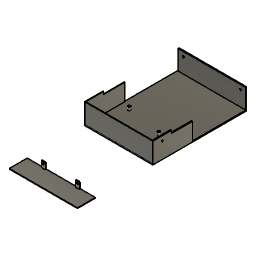
BakjeCNCPCBShizzle v1 (Autodesk Fusion 360 design; units mm, degrees)
Autodesk Fusion 360 part; units mm, degrees
sketch "Sketch1" plane through (0, 0, 0) normal (0, 0, 1) x (1, 0, 0)
  line L0 (0, 142.5) -> (129, 142.5)
  line L1 (129, 142.5) -> (129, 217.5)
  line L2 (129, 217.5) -> (0, 217.5)
  line L3 (0, 217.5) -> (0, 142.5)
  line L4 (0, 0) -> (1, 0)
  line L5 (1, 217.5) -> (0, 217.5)
  line L6 (129, 217.5) -> (0, 217.5)
  line L7 (0, 217.5) -> (0, 320)
  line L8 (0, 320) -> (129, 320)
  line L9 (129, 320) -> (129, 217.5)
  line L10 (0, 217.5) -> (1, 217.5)
  line L11 (1, 217.5) -> (1, 142.5)
  line L12 (1, 142.5) -> (0, 142.5)
  line L13 (0, 142.5) -> (0, 217.5)
  line L14 (129, 142.5) -> (127, 142.5)
  line L15 (127, 142.5) -> (127, 217.5)
  line L16 (127, 217.5) -> (129, 217.5)
  line L17 (129, 217.5) -> (129, 142.5)
  line L18 (0, 320) -> (129, 320)
  line L19 (129, 320) -> (129, 318)
  line L20 (129, 318) -> (0, 318)
  line L21 (0, 318) -> (0, 320)
  line L22 (1, 142.5) -> (127, 142.5)
  line L23 (127, 142.5) -> (127, 143.5)
  line L24 (127, 143.5) -> (1, 143.5)
  line L25 (1, 143.5) -> (1, 142.5)
  line L26 (0, 320) -> (1, 320)
  line L27 (1, 320) -> (1, 283)
  line L28 (1, 283) -> (0, 283)
  line L29 (0, 283) -> (0, 320)
  line L30 (0, 217.5) -> (0, 177.5)
  line L31 (0, 177.5) -> (1, 177.5)
  line L32 (1, 177.5) -> (129, 177.5)
  dimension "d2" = 142.5
  dimension "d3" = 129
  dimension "d4" = 75
  dimension "d5" = 1
  dimension "d6" = 129
  dimension "d7" = 102.5
  dimension "d8" = 1
  dimension "d9" = 2
  dimension "d10" = 2
  dimension "d11" = 1
  dimension "d12" = 1
  dimension "d29" = 40
  constraint horizontal L0
  constraint vertical L1
  constraint horizontal L2
  constraint vertical L3
  constraint horizontal L4
  constraint horizontal L5
  constraint coincident L2 L5.start
  constraint coincident L4.start origin
  constraint horizontal L6
  constraint vertical L7
  constraint horizontal L8
  constraint vertical L9
  constraint horizontal L10
  constraint vertical L11
  constraint horizontal L12
  constraint vertical L13
  constraint horizontal L14
  constraint vertical L15
  constraint horizontal L16
  constraint vertical L17
  constraint coincident L6 L15.end
  constraint horizontal L18
  constraint vertical L19
  constraint horizontal L20
  constraint vertical L21
  constraint coincident L9 L19.end
  constraint horizontal L22
  constraint vertical L23
  constraint horizontal L24
  constraint vertical L25
  constraint horizontal L26
  constraint vertical L27
  constraint horizontal L28
  constraint vertical L29
  constraint coincident L3 L30.end
  constraint coincident L11 L31.end
  constraint perpendicular L11 L31
  constraint coincident L17 L32.end
  constraint perpendicular L17 L32
  measures "d2" distance of L4.start L0.start
  measures "d3" distance of L0.start L0.end
  measures "d4" distance of L0.start L2.end
  measures "d5" distance of L4.start L4.end
  measures "d6" distance of L1.end L2.end
  measures "d7" distance of L1.end L8.end
  measures "d8" distance of L2.end L5.start
  measures "d9" distance of L0.end L14.end
  measures "d10" distance of L7.end L20.end
  measures "d11" distance of L11.end L24.end
  measures "d12" distance of L7.end L26.end
  measures "d29" distance of L2.end L30.end
extrude "Extrude1" add sketch "Sketch1" along normal blind 39 contours L0 L3 L11 L12 L13 L25 L31 | L0 L11 L15 L22 L23 L24 L25 | L0 L1 L14 L15 L17 L23 L32 | L8 L9 L18 L19 L20 L27 makes body 1 at (43.6667, 320, 13) makes body 2 at (43, 142.5, 26)
extrude "Extrude2" add sketch "Sketch1" along normal blind 2 contours L11 L15 L24 L32 | L2 L5 L6 L7 L9 L10 L16 L20 L27 L28 | L2 L6 L11 L15 L32 | L7 L20 L27 L28 L29 bodies 1 2
sketch "Sketch2" plane through (0, 318, 0) normal (0, -1, 0) x (1, 0, 0)
  line L0 (1, 2) -> (129, 2)
  line L1 (129, 2) -> (129, 39)
  line L2 (129, 39) -> (1, 39)
  line L3 (1, 39) -> (1, 2)
  line L4 (1, 39) -> (129, 39)
  line L5 (1, 39) -> (11, 39)
  line L6 (11, 39) -> (11, 30.25)
  circle A0 centre (11, 30.25) radius 1.75
  line L7 (129, 39) -> (119, 39)
  line L8 (119, 39) -> (119, 30.25)
  circle A1 centre (119, 30.25) radius 1.75
  dimension "d17" = 10
  dimension "d18" = 8.75
  dimension "d19" = 3.5
  dimension "d20" = 10
  dimension "d21" = 8.75
  dimension "d22" = 3.5
  constraint coincident L2.end L3.start
  constraint coincident L1.end L2.start
  constraint perpendicular L3 L5
  constraint perpendicular L5 L6
  constraint coincident L6.end A0.centre
  constraint perpendicular L1 L7
  constraint perpendicular L7 L8
  constraint coincident L8.end A1.centre
  measures "d17" distance of L2.end L5.end
  measures "d18" distance of L5.end L6.end
  measures "d19" diameter of A0
  measures "d20" distance of L1.end L7.end
  measures "d21" distance of L7.end L8.end
  measures "d22" diameter of A1
extrude "Extrude3" cut sketch "Sketch2" against normal blind 90 contours A0 | A1 bodies 1
sketch "Sketch3" plane through (127, 0, 0) normal (-1, 0, 0) x (0, -1, 0)
  line L0 (-177.5, 2) -> (-143.5, 2)
  line L1 (-143.5, 2) -> (-143.5, 39)
  line L2 (-143.5, 39) -> (-177.5, 39)
  line L3 (-177.5, 39) -> (-143.5, 39)
  line L4 (-160.5, 39) -> (-160.5, 30.25)
  circle A0 centre (-160.5, 30.25) radius 1.75
  line L5 (-177.5, 39) -> (-177.5, 2)
  dimension "d25" = 8.75
  dimension "d26" = 3.5
  constraint coincident L2.end L3.start
  constraint coincident L1.end L2.start
  constraint midpoint L3 L4.start
  constraint perpendicular L3 L4
  constraint coincident L4.end A0.centre
  measures "d25" distance of L4.start L4.end
  measures "d26" diameter of A0
extrude "Extrude4" cut sketch "Sketch3" against normal blind 43 contours A0 bodies 1
sketch "Sketch4" plane through (0, 0, 2) normal (0, 0, 1) x (-1, 0, 0)
  line L0 (-129, -318) -> (-1, -318)
  line L1 (-1, -318) -> (0, -318)
  line L2 (0, -318) -> (0, -217.5)
  line L3 (-129, -217.5) -> (-129, -318)
  line L4 (0, -217.5) -> (-1, -217.5)
  line L5 (-127, -217.5) -> (-129, -217.5)
  line L6 (-1, -217.5) -> (-1, -177.5)
  line L7 (-1, -177.5) -> (-1, -143.5)
  line L8 (-1, -143.5) -> (-127, -143.5)
  line L9 (-127, -143.5) -> (-127, -177.5)
  line L10 (-127, -177.5) -> (-127, -217.5)
extrude "Extrude5" add sketch "Sketch1" along normal blind 34 contours L2 L3 L5 L6 L10 L11 L13 L30 L31 | L1 L2 L6 L15 L16 L17 L32 bodies 1
sketch "Sketch5" plane through (0, 0, 0) normal (0, 0, 1) x (1, 0, 0)
  line L0 (0, 0) -> (129, 0)
  line L1 (129, 0) -> (129, 34)
  line L2 (129, 34) -> (0, 34)
  line L3 (0, 34) -> (0, 0)
  line L4 (0, 34) -> (129, 34)
  line L5 (64.5, 34) -> (0, 34)
  line L6 (64.5, 34) -> (129, 34)
  line L7 (32.25, 34) -> (32.25, 33)
  line L8 (96.75, 34) -> (96.75, 33)
  line L9 (36, 34) -> (28.5, 34)
  line L10 (28.5, 34) -> (28.5, 32)
  line L11 (28.5, 32) -> (36, 32)
  line L12 (36, 32) -> (36, 34)
  line L13 (36, 34) -> (28.5, 32) construction
  line L14 (28.5, 34) -> (36, 32) construction
  line L15 (100.5, 32) -> (93, 32)
  line L16 (93, 32) -> (93, 34)
  line L17 (93, 34) -> (100.5, 34)
  line L18 (100.5, 34) -> (100.5, 32)
  line L19 (100.5, 32) -> (93, 34) construction
  line L20 (93, 32) -> (100.5, 34) construction
  point P0 (32.25, 33)
  point P1 (96.75, 33)
  dimension "d32" = 129
  dimension "d33" = 34
  dimension "d34" = 1
  dimension "d35" = 1
  dimension "d36" = 7.5
  dimension "d37" = 2
  dimension "d38" = 7.5
  dimension "d39" = 2
  constraint horizontal L0
  constraint vertical L1
  constraint horizontal L2
  constraint vertical L3
  constraint coincident L0.start L3.end
  constraint midpoint L2 L5.start
  constraint midpoint L5 L7.start
  constraint perpendicular L4 L7
  constraint midpoint L6 L8.start
  constraint vertical L8
  constraint horizontal L9
  constraint perpendicular L9 L10
  constraint parallel L9 L11
  constraint parallel L10 L12
  constraint coincident L13 P0
  constraint coincident L14 P0
  constraint coincident P0 L7.end
  constraint horizontal L15
  constraint perpendicular L15 L16
  constraint parallel L15 L17
  constraint parallel L16 L18
  constraint coincident L19 P1
  constraint coincident L20 P1
  constraint coincident P1 L8.end
  measures "d32" distance of L0.start L0.end
  measures "d33" distance of L0.start L2.end
  measures "d34" distance of L7.start P0
  measures "d35" distance of L8.start P1
  measures "d36" distance of L10.end L11.end
  measures "d37" distance of L9.end L10.end
  measures "d38" distance of L16.end L17.end
  measures "d39" distance of L15.end L16.end
extrude "Extrude6" add sketch "Sketch5" along normal blind 1 separate body contours L0 L1 L2 L3 L4 L5 L6 L10 L11 L12 L15 L16 L18 makes body 3
extrude "Extrude7" add sketch "Sketch5" along normal blind 12.25 contours L2 L4 L5 L9 L10 L11 L12 | L2 L4 L6 L15 L16 L17 L18 bodies 3
sketch "Sketch6" plane through (0, 32, 0) normal (0, -1, 0) x (1, 0, 0)
  line L0 (28.5, 1) -> (36, 1)
  line L1 (36, 1) -> (36, 12.25)
  line L2 (36, 12.25) -> (28.5, 12.25)
  line L3 (28.5, 12.25) -> (28.5, 1)
  line L4 (32.25, 1) -> (32.25, 8.75)
  circle A0 centre (32.25, 8.75) radius 1.75
  dimension "d44" = 7.75
  dimension "d45" = 3.5
  constraint midpoint L0 L4.start
  constraint perpendicular L0 L4
  constraint coincident L4.end A0.centre
  measures "d44" distance of L4.start L4.end
  measures "d45" diameter of A0
sketch "Sketch7" plane through (0, 32, 0) normal (0, -1, 0) x (1, 0, 0)
  line L0 (93, 1) -> (100.5, 1)
  line L1 (100.5, 1) -> (100.5, 12.25)
  line L2 (100.5, 12.25) -> (93, 12.25)
  line L3 (93, 12.25) -> (93, 1)
  line L4 (96.75, 1) -> (96.75, 8.75)
  circle A0 centre (96.75, 8.75) radius 1.75
  dimension "d46" = 7.75
  dimension "d47" = 3.5
  constraint midpoint L0 L4.start
  constraint perpendicular L0 L4
  constraint coincident L4.end A0.centre
  measures "d46" distance of L4.start L4.end
  measures "d47" diameter of A0
extrude "Extrude8" cut sketch "Sketch6" sketch "Sketch7" against normal blind 15 contours A0 of sketch 2 contours A0 bodies 3
sketch "Sketch8" plane through (0, 0, 2) normal (0, 0, 1) x (-1, 0, 0)
  line L0 (-127, -217.5) -> (-129, -217.5)
  line L1 (-129, -217.5) -> (-129, -318)
  line L2 (-129, -318) -> (-1, -318)
  line L3 (-1, -318) -> (0, -318)
  line L4 (0, -318) -> (0, -217.5)
  line L5 (0, -217.5) -> (-1, -217.5)
  line L6 (-1, -217.5) -> (-1, -143.5)
  line L7 (-1, -143.5) -> (-127, -143.5)
  line L8 (-127, -143.5) -> (-127, -217.5)
  line L9 (-127, -217.5) -> (-1, -217.5)
  line L10 (-64, -217.5) -> (-64, -143.5)
  line L11 (-64, -217.5) -> (-127, -217.5)
  line L12 (-95.5, -217.5) -> (-95.5, -143.5)
  line L13 (-127, -217.5) -> (-95.5, -143.5)
  line L14 (-100.25, -159.5) -> (-122.25, -159.5)
  line L15 (-122.25, -159.5) -> (-122.25, -201.5)
  line L16 (-122.25, -201.5) -> (-100.25, -201.5)
  line L17 (-100.25, -201.5) -> (-100.25, -159.5)
  line L18 (-100.25, -159.5) -> (-122.25, -201.5) construction
  line L19 (-122.25, -159.5) -> (-100.25, -201.5) construction
  line L20 (-64, -143.5) -> (-95.5, -217.5)
  line L21 (-68.75, -201.5) -> (-90.75, -201.5)
  line L22 (-90.75, -201.5) -> (-90.75, -159.5)
  line L23 (-90.75, -159.5) -> (-68.75, -159.5)
  line L24 (-68.75, -159.5) -> (-68.75, -201.5)
  line L25 (-68.75, -201.5) -> (-90.75, -159.5) construction
  line L26 (-90.75, -201.5) -> (-68.75, -159.5) construction
  line L27 (-100.25, -159.5) -> (-100.25, -166)
  line L28 (-100.25, -166) -> (-103.25, -166)
  circle A0 centre (-103.25, -166) radius 1.5
  line L29 (-122.25, -201.5) -> (-122.25, -195)
  line L30 (-122.25, -195) -> (-119.25, -195)
  circle A1 centre (-103.25, -166) radius 2.5
  circle A2 centre (-119.25, -195) radius 1.5
  circle A3 centre (-119.25, -195) radius 2.5
  line L31 (-68.75, -159.5) -> (-68.75, -166)
  line L32 (-68.75, -166) -> (-71.75, -166)
  circle A4 centre (-71.75, -166) radius 1.5
  circle A5 centre (-71.75, -166) radius 2.5
  line L33 (-90.75, -201.5) -> (-90.75, -195)
  line L34 (-90.75, -195) -> (-87.75, -195)
  circle A6 centre (-87.75, -195) radius 1.5
  circle A7 centre (-87.75, -195) radius 2.5
  line L35 (-64, -217.5) -> (-1, -143.5)
  line L36 (-16, -211) -> (-49, -211)
  line L37 (-49, -211) -> (-49, -150)
  line L38 (-49, -150) -> (-16, -150)
  line L39 (-16, -150) -> (-16, -211)
  line L40 (-16, -211) -> (-49, -150) construction
  line L41 (-49, -211) -> (-16, -150) construction
  line L42 (-49, -150) -> (-46.5, -150)
  line L43 (-46.5, -150) -> (-46.5, -152.5)
  line L44 (-46.5, -152.5) -> (-49, -152.5)
  line L45 (-49, -152.5) -> (-49, -150)
  line L46 (-16, -211) -> (-18.5, -211)
  line L47 (-18.5, -211) -> (-18.5, -208.5)
  line L48 (-18.5, -208.5) -> (-16, -208.5)
  line L49 (-16, -208.5) -> (-16, -211)
  circle A8 centre (-46.5, -152.5) radius 1.5
  circle A9 centre (-18.5, -208.5) radius 1.5
  circle A10 centre (-46.5, -152.5) radius 2.5
  circle A11 centre (-18.5, -208.5) radius 2.5
  point P0 (-111.25, -180.5)
  point P1 (-79.75, -180.5)
  point P2 (-32.5, -180.5)
  dimension "d50" = 22
  dimension "d51" = 42
  dimension "d52" = 22
  dimension "d53" = 42
  dimension "d54" = 6.5
  dimension "d55" = 3
  dimension "d56" = 3
  dimension "d57" = 6.5
  dimension "d58" = 3
  dimension "d59" = 5
  dimension "d60" = 3
  dimension "d61" = 5
  dimension "d62" = 6.5
  dimension "d63" = 3
  dimension "d64" = 3
  dimension "d65" = 5
  dimension "d66" = 6.5
  dimension "d67" = 3
  dimension "d68" = 3
  dimension "d69" = 5
  dimension "d70" = 33
  dimension "d71" = 61
  dimension "d72" = 2.5
  dimension "d73" = 2.5
  dimension "d74" = 2.5
  dimension "d75" = 2.5
  dimension "d76" = 3
  dimension "d77" = 3
  dimension "d78" = 5
  dimension "d79" = 5
  constraint coincident L0.start L8.end
  constraint coincident L5.end L6.start
  constraint midpoint L9 L10.start
  constraint midpoint L7 L10.end
  constraint midpoint L11 L12.start
  constraint coincident L7 L12.end
  constraint perpendicular L7 L12
  constraint horizontal L14
  constraint perpendicular L14 L15
  constraint parallel L14 L16
  constraint parallel L15 L17
  constraint coincident L18 P0
  constraint coincident L19 P0
  constraint midpoint L13 P0
  constraint horizontal L21
  constraint perpendicular L21 L22
  constraint parallel L21 L23
  constraint parallel L22 L24
  constraint coincident L25 P1
  constraint coincident L26 P1
  constraint midpoint L20 P1
  constraint perpendicular L14 L27
  constraint perpendicular L27 L28
  constraint coincident L28.end A0.centre
  constraint perpendicular L16 L29
  constraint perpendicular L29 L30
  constraint concentric A0 A1
  constraint coincident L30.end A2.centre
  constraint concentric A2 A3
  constraint coincident L24 L31.end
  constraint perpendicular L31 L32
  constraint coincident L32.end A4.centre
  constraint concentric A4 A5
  constraint perpendicular L21 L33
  constraint perpendicular L22 L34
  constraint coincident L34.end A6.centre
  constraint concentric A6 A7
  constraint coincident L6.end L7.start
  constraint horizontal L36
  constraint perpendicular L36 L37
  constraint parallel L36 L38
  constraint parallel L37 L39
  constraint coincident L40 P2
  constraint coincident L41 P2
  constraint midpoint L35 P2
  constraint horizontal L42
  constraint vertical L43
  constraint horizontal L44
  constraint vertical L45
  constraint horizontal L46
  constraint vertical L47
  constraint horizontal L48
  constraint vertical L49
  constraint coincident L43.end L44.start
  constraint coincident L47.end L48.start
  constraint concentric A8 A10
  constraint concentric A9 A11
  measures "d50" distance of L15.end L16.end
  measures "d51" distance of L14.end L15.end
  measures "d52" distance of L22.end L23.end
  measures "d53" distance of L21.end L22.end
  measures "d54" distance of L14.start L27.end
  measures "d55" distance of L27.end L28.end
  measures "d56" diameter of A0
  measures "d57" distance of L15.end L29.end
  measures "d58" distance of L29.end L30.end
  measures "d59" diameter of A1
  measures "d60" diameter of A2
  measures "d61" diameter of A3
  measures "d62" distance of L23.end L31.end
  measures "d63" distance of L31.end L32.end
  measures "d64" diameter of A4
  measures "d65" diameter of A5
  measures "d66" distance of L21.end L33.end
  measures "d67" distance of L33.end L34.end
  measures "d68" diameter of A6
  measures "d69" diameter of A7
  measures "d70" distance of L37.end L38.end
  measures "d71" distance of L36.end L37.end
  measures "d72" distance of L37.end L42.end
  measures "d73" distance of L37.end L44.end
  measures "d74" distance of L36.start L46.end
  measures "d75" distance of L36.start L48.end
  measures "d76" diameter of A8
  measures "d77" diameter of A9
  measures "d78" diameter of A10
  measures "d79" diameter of A11
extrude "Extrude9" add sketch "Sketch8" along normal blind 6 contours L13 A3 | L13 A3 | L20 A7 | L20 A7 | L13 A1 | L13 A1 | L43 L44 A8 A10 | L43 L44 A8 A10 | L20 A5 | L20 A5 | L47 L48 A9 A11 | L47 L48 A9 A11 bodies 1
equation "d18 = 7 mm + ( ( 3.5 / 2 ) * 1 mm )"
equation "d42 = 8.75 mm + 3.5 mm"
equation "d54 = 5 mm + 1.5 mm"
